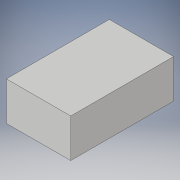
# Autodesk Inventor part: Arduino
Saved by Autodesk Inventor 2019.5 (Build 235369000, 369)
## iProperties
Created: 2021-09-30
Part Number: Arduino
Material: Generisch
Document SubType Name: Modeling
Designer: mritt
Density: 1 g/cm^3
Appearance: Vorgabe
Author: mritt
Autodesk Inventor part; units mm, degrees
ref_plane "YZ Plane" through (0, 0, 0) normal (1, 0, 0) x (0, 1, 0)
ref_plane "XZ Plane" through (0, 0, 0) normal (0, 1, 0) x (-1, 0, 0)
ref_plane "XY Plane" through (0, 0, 0) normal (0, 0, 1) x (1, 0, 0)
sketch "Skizze1" plane through (0, 0, 0) normal (0, 1, 0) x (-1, 0, 0)
  line L0 (99.2126, -64.252) -> (49.2126, -64.252)
  line L1 (49.2126, -64.252) -> (49.2126, -144.252)
  line L2 (49.2126, -144.252) -> (99.2126, -144.252)
  line L3 (99.2126, -144.252) -> (99.2126, -64.252)
  point P0 (0, 0)
  dimension "d0" = 80
  dimension "d1" = 50
  constraints: 8 end point, 2 parallel, 1 horizontal, 1 perpendicular
  measures "d0" distance of L2.end L0.start
  measures "d1" distance of L1.end L2.end
extrude "Extrusion1" add sketch "Skizze1" along normal blind 30
